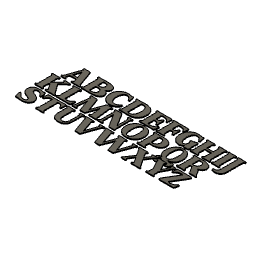
alphabet v02 (Autodesk Fusion 360 design; units mm, degrees)
Autodesk Fusion 360 part; units mm, degrees
(part 1 of 8)
sketch "Sketch1" plane through (0, 0, 0) normal (0, 0, 1) x (1, 0, 0)
  line L0 (-281.2306, -198.9387) -> (-284.5117, -189.696)
  line L1 (-284.5117, -189.696) -> (-287.7576, -198.9035)
  line L2 (-287.7576, -198.9035) -> (-281.2306, -198.9387)
  spline S0 degree 3 poles (-289.8743, -204.8301) (-290.4035, -206.2765) (-288.1104, -206.2412) (-288.1104, -206.7704) knots 0 0 0 0 1 1 1 1
  spline S1 degree 3 poles (-288.1104, -206.7704) (-288.1104, -207.1937) (-288.4985, -208.0051) (-288.7807, -207.9699) knots 0 0 0 0 1 1 1 1
  spline S2 degree 3 poles (-288.7807, -207.9699) (-289.3099, -207.8993) (-290.3686, -207.864) (-291.4269, -207.864) knots 0 0 0 0 1 1 1 1
  spline S3 degree 3 poles (-291.4269, -207.864) (-292.4852, -207.864) (-293.5436, -207.8993) (-294.0727, -207.9699) knots 0 0 0 0 1 1 1 1
  spline S4 degree 3 poles (-294.0727, -207.9699) (-294.3902, -208.0051) (-294.743, -207.1937) (-294.743, -206.7704) knots 0 0 0 0 1 1 1 1
  spline S5 degree 3 poles (-294.743, -206.7704) (-294.743, -206.2412) (-293.1555, -206.2412) (-292.6616, -204.8301) knots 0 0 0 0 1 1 1 1
  line L3 (-292.6616, -204.8301) -> (-286.0992, -186.4151)
  spline S6 degree 3 poles (-286.0992, -186.4151) (-286.699, -185.9565) (-287.4045, -185.7801) (-287.4045, -185.4274) knots 0 0 0 0 1 1 1 1
  spline S7 degree 3 poles (-287.4045, -185.4274) (-287.4045, -185.004) (-287.0168, -184.2244) (-286.7346, -184.2632) knots 0 0 0 0 1 1 1 1
  spline S8 degree 3 poles (-286.7346, -184.2632) (-284.2295, -184.4749) (-281.5484, -184.2632) (-280.3486, -184.2632) knots 0 0 0 0 1 1 1 1
  spline S9 degree 3 poles (-280.3486, -184.2632) (-279.1492, -184.2632) (-278.7964, -184.4749) (-278.5847, -185.0746) knots 0 0 0 0 1 1 1 1
  line L4 (-278.5847, -185.0746) -> (-271.5641, -204.8301)
  spline S10 degree 3 poles (-271.5641, -204.8301) (-271.0702, -206.2765) (-269.4827, -206.2412) (-269.4827, -206.7704) knots 0 0 0 0 1 1 1 1
  spline S11 degree 3 poles (-269.4827, -206.7704) (-269.4827, -207.1937) (-269.8355, -207.9699) (-270.1174, -207.9699) knots 0 0 0 0 1 1 1 1
  spline S12 degree 3 poles (-270.1174, -207.9699) (-271.5288, -207.8993) (-273.3633, -207.864) (-275.1981, -207.864) knots 0 0 0 0 1 1 1 1
  spline S13 degree 3 poles (-275.1981, -207.864) (-277.0325, -207.864) (-278.8317, -207.8993) (-280.2428, -207.9699) knots 0 0 0 0 1 1 1 1
  spline S14 degree 3 poles (-280.2428, -207.9699) (-280.525, -207.9699) (-280.9134, -207.1937) (-280.9134, -206.7704) knots 0 0 0 0 1 1 1 1
  spline S15 degree 3 poles (-280.9134, -206.7704) (-280.9134, -206.2412) (-278.6553, -206.2765) (-279.1492, -204.8301) knots 0 0 0 0 1 1 1 1
  line L5 (-279.1492, -204.8301) -> (-280.3842, -201.4082)
  line L6 (-280.3842, -201.4082) -> (-288.6749, -201.4787)
  line L7 (-288.6749, -201.4787) -> (-289.8743, -204.8301)
  spline S16 degree 3 poles (-259.2536, -204.7243) (-259.2536, -205.571) (-257.4897, -205.5357) (-256.8194, -205.5357) knots 0 0 0 0 1 1 1 1
  spline S17 degree 3 poles (-256.8194, -205.5357) (-253.2916, -205.5357) (-251.351, -204.0187) (-251.351, -201.1965) knots 0 0 0 0 1 1 1 1
  spline S18 degree 3 poles (-251.351, -201.1965) (-251.351, -198.3743) (-253.256, -196.8221) (-256.6787, -196.8221) knots 0 0 0 0 1 1 1 1
  line L8 (-256.6787, -196.8221) -> (-259.2536, -196.8221)
  line L9 (-259.2536, -196.8221) -> (-259.2536, -204.7243)
  spline S19 degree 3 poles (-256.9605, -194.3526) (-254.103, -194.3526) (-252.4093, -192.9415) (-252.4093, -190.5426) knots 0 0 0 0 1 1 1 1
  spline S20 degree 3 poles (-252.4093, -190.5426) (-252.4093, -188.179) (-254.103, -186.7326) (-256.9605, -186.7326) knots 0 0 0 0 1 1 1 1
  spline S21 degree 3 poles (-256.9605, -186.7326) (-258.76, -186.7326) (-259.2536, -186.6974) (-259.2536, -187.544) knots 0 0 0 0 1 1 1 1
  line L10 (-259.2536, -187.544) -> (-259.2536, -194.3526)
  line L11 (-259.2536, -194.3526) -> (-256.9605, -194.3526)
  spline S22 degree 3 poles (-243.6248, -201.3729) (-243.6248, -205.7121) (-247.5763, -208.0051) (-255.1614, -208.0051) knots 0 0 0 0 1 1 1 1
  spline S23 degree 3 poles (-255.1614, -208.0051) (-258.8659, -208.0051) (-260.4883, -207.8993) (-262.9934, -207.8993) knots 0 0 0 0 1 1 1 1
  spline S24 degree 3 poles (-262.9934, -207.8993) (-264.5456, -207.8993) (-266.2393, -207.9346) (-267.6504, -208.0051) knots 0 0 0 0 1 1 1 1
  spline S25 degree 3 poles (-267.6504, -208.0051) (-267.9326, -208.0404) (-268.321, -207.2643) (-268.321, -206.841) knots 0 0 0 0 1 1 1 1
  spline S26 degree 3 poles (-268.321, -206.841) (-268.321, -206.2765) (-266.3804, -206.3824) (-266.3804, -204.9007) knots 0 0 0 0 1 1 1 1
  line L12 (-266.3804, -204.9007) -> (-266.3804, -187.3676)
  spline S27 degree 3 poles (-266.3804, -187.3676) (-266.3804, -185.886) (-268.321, -185.9918) (-268.321, -185.4274) knots 0 0 0 0 1 1 1 1
  spline S28 degree 3 poles (-268.321, -185.4274) (-268.321, -185.004) (-267.9326, -184.2244) (-267.6504, -184.2632) knots 0 0 0 0 1 1 1 1
  spline S29 degree 3 poles (-267.6504, -184.2632) (-266.2393, -184.3337) (-264.5456, -184.369) (-262.9934, -184.369) knots 0 0 0 0 1 1 1 1
  spline S30 degree 3 poles (-262.9934, -184.369) (-260.4883, -184.369) (-258.8659, -184.2632) (-255.1614, -184.2632) knots 0 0 0 0 1 1 1 1
  spline S31 degree 3 poles (-255.1614, -184.2632) (-248.2462, -184.2632) (-244.6832, -186.4857) (-244.6832, -190.2957) knots 0 0 0 0 1 1 1 1
  spline S32 degree 3 poles (-244.6832, -190.2957) (-244.6832, -192.5182) (-245.8826, -194.2115) (-248.2818, -195.3404) knots 0 0 0 0 1 1 1 1
  spline S33 degree 3 poles (-248.2818, -195.3404) (-245.2476, -196.5046) (-243.6248, -198.586) (-243.6248, -201.3729) knots 0 0 0 0 1 1 1 1
  spline S34 degree 3 poles (-220.7302, -201.0201) (-220.5189, -200.7732) (-219.4606, -201.0907) (-219.4606, -201.3729) knots 0 0 0 0 1 1 1 1
  spline S35 degree 3 poles (-219.4606, -201.3729) (-219.4606, -202.5371) (-222.4945, -208.3579) (-229.762, -208.3579) knots 0 0 0 0 1 1 1 1
  spline S36 degree 3 poles (-229.762, -208.3579) (-236.5713, -208.3579) (-241.475, -203.2426) (-241.475, -196.1518) knots 0 0 0 0 1 1 1 1
  spline S37 degree 3 poles (-241.475, -196.1518) (-241.475, -188.9904) (-236.4655, -183.9104) (-229.4445, -183.9104) knots 0 0 0 0 1 1 1 1
  spline S38 degree 3 poles (-229.4445, -183.9104) (-226.622, -183.9104) (-225.3167, -184.616) (-224.1173, -184.616) knots 0 0 0 0 1 1 1 1
  spline S39 degree 3 poles (-224.1173, -184.616) (-223.2353, -184.616) (-222.9531, -184.2632) (-222.3883, -184.2632) knots 0 0 0 0 1 1 1 1
  spline S40 degree 3 poles (-222.3883, -184.2632) (-221.93, -184.2632) (-221.6478, -184.6865) (-221.4714, -185.3568) knots 0 0 0 0 1 1 1 1
  spline S41 degree 3 poles (-221.4714, -185.3568) (-221.33, -185.886) (-220.5539, -190.3662) (-220.5539, -190.6485) knots 0 0 0 0 1 1 1 1
  spline S42 degree 3 poles (-220.5539, -190.6485) (-220.5539, -190.9307) (-221.33, -191.6715) (-221.7536, -191.6715) knots 0 0 0 0 1 1 1 1
  spline S43 degree 3 poles (-221.7536, -191.6715) (-222.3883, -191.6715) (-224.1525, -186.4504) (-228.4215, -186.4504) knots 0 0 0 0 1 1 1 1
  spline S44 degree 3 poles (-228.4215, -186.4504) (-231.7376, -186.4504) (-233.7135, -189.6254) (-233.7135, -194.9171) knots 0 0 0 0 1 1 1 1
  spline S45 degree 3 poles (-233.7135, -194.9171) (-233.7135, -200.9143) (-231.1735, -204.3715) (-226.9398, -204.3715) knots 0 0 0 0 1 1 1 1
  spline S46 degree 3 poles (-226.9398, -204.3715) (-224.6464, -204.3715) (-222.812, -203.3485) (-220.7302, -201.0201) knots 0 0 0 0 1 1 1 1
  spline S47 degree 3 poles (-206.8319, -186.7326) (-208.5958, -186.7326) (-209.1249, -186.6621) (-209.1249, -187.544) knots 0 0 0 0 1 1 1 1
  line L13 (-209.1249, -187.544) -> (-209.1249, -204.689)
  spline S48 degree 3 poles (-209.1249, -204.689) (-209.1249, -205.571) (-207.3258, -205.5004) (-206.7962, -205.5004) knots 0 0 0 0 1 1 1 1
  spline S49 degree 3 poles (-206.7962, -205.5004) (-202.7746, -205.5004) (-200.5874, -202.3607) (-200.5874, -196.1165) knots 0 0 0 0 1 1 1 1
  spline S50 degree 3 poles (-200.5874, -196.1165) (-200.5874, -189.8724) (-202.7746, -186.7326) (-206.8319, -186.7326) knots 0 0 0 0 1 1 1 1
  spline S51 degree 3 poles (-212.8294, -207.8993) (-214.3817, -207.8993) (-216.1103, -207.9346) (-217.5214, -208.0051) knots 0 0 0 0 1 1 1 1
  spline S52 degree 3 poles (-217.5214, -208.0051) (-217.8036, -208.0051) (-218.1564, -207.2643) (-218.1564, -206.841) knots 0 0 0 0 1 1 1 1
  spline S53 degree 3 poles (-218.1564, -206.841) (-218.1564, -206.2765) (-216.2514, -206.3824) (-216.2514, -204.8654) knots 0 0 0 0 1 1 1 1
  line L14 (-216.2514, -204.8654) -> (-216.2514, -187.3676)
  spline S54 degree 3 poles (-216.2514, -187.3676) (-216.2514, -185.886) (-218.192, -185.9918) (-218.192, -185.4274) knots 0 0 0 0 1 1 1 1
  spline S55 degree 3 poles (-218.192, -185.4274) (-218.192, -185.004) (-217.8036, -184.2244) (-217.5214, -184.2632) knots 0 0 0 0 1 1 1 1
  spline S56 degree 3 poles (-217.5214, -184.2632) (-216.1103, -184.3337) (-214.4169, -184.369) (-212.8294, -184.369) knots 0 0 0 0 1 1 1 1
  spline S57 degree 3 poles (-212.8294, -184.369) (-210.3596, -184.369) (-208.9133, -184.2632) (-205.2087, -184.2632) knots 0 0 0 0 1 1 1 1
  spline S58 degree 3 poles (-205.2087, -184.2632) (-197.8001, -184.2632) (-192.8259, -189.0257) (-192.8259, -196.1518) knots 0 0 0 0 1 1 1 1
  spline S59 degree 3 poles (-192.8259, -196.1518) (-192.8259, -203.2779) (-197.7648, -208.0051) (-205.2087, -208.0051) knots 0 0 0 0 1 1 1 1
  spline S60 degree 3 poles (-205.2087, -208.0051) (-208.9133, -207.9699) (-210.3596, -207.8993) (-212.8294, -207.8993) knots 0 0 0 0 1 1 1 1
  line L15 (-182.4916, -194.4232) -> (-180.0222, -194.3526)
  spline S61 degree 3 poles (-180.0222, -194.3526) (-177.1294, -194.2821) (-177.3411, -190.6485) (-176.2827, -190.6485) knots 0 0 0 0 1 1 1 1
  spline S62 degree 3 poles (-176.2827, -190.6485) (-175.8594, -190.6485) (-175.0833, -191.0365) (-175.0833, -191.3187) knots 0 0 0 0 1 1 1 1
  spline S63 degree 3 poles (-175.0833, -191.3187) (-175.2597, -194.2115) (-175.2597, -197.1043) (-175.0833, -199.9971) knots 0 0 0 0 1 1 1 1
  spline S64 degree 3 poles (-175.0833, -199.9971) (-175.0833, -200.2793) (-175.8594, -200.6674) (-176.2827, -200.6674) knots 0 0 0 0 1 1 1 1
  spline S65 degree 3 poles (-176.2827, -200.6674) (-177.3411, -200.6674) (-177.1294, -197.0337) (-180.0222, -196.9632) knots 0 0 0 0 1 1 1 1
  line L16 (-180.0222, -196.9632) -> (-182.4916, -196.8926)
  line L17 (-182.4916, -196.8926) -> (-182.4916, -204.2657)
  spline S66 degree 3 poles (-182.4916, -204.2657) (-182.4916, -205.1829) (-182.1036, -205.4299) (-179.9163, -205.4299) knots 0 0 0 0 1 1 1 1
  spline S67 degree 3 poles (-179.9163, -205.4299) (-173.5311, -205.4299) (-172.508, -201.3024) (-171.8377, -201.3024) knots 0 0 0 0 1 1 1 1
  spline S68 degree 3 poles (-171.8377, -201.3024) (-171.4144, -201.3024) (-170.6383, -201.6551) (-170.6383, -201.9374) knots 0 0 0 0 1 1 1 1
  spline S69 degree 3 poles (-170.6383, -201.9374) (-170.6383, -202.2196) (-171.5908, -206.4529) (-171.7319, -206.9821) knots 0 0 0 0 1 1 1 1
  spline S70 degree 3 poles (-171.7319, -206.9821) (-171.9788, -207.7935) (-172.2611, -208.0404) (-173.0019, -208.0051) knots 0 0 0 0 1 1 1 1
  spline S71 degree 3 poles (-173.0019, -208.0051) (-175.4713, -207.9346) (-178.6816, -207.8993) (-181.9272, -207.8993) knots 0 0 0 0 1 1 1 1
  spline S72 degree 3 poles (-181.9272, -207.8993) (-185.1371, -207.8993) (-188.3827, -207.9346) (-190.8524, -208.0051) knots 0 0 0 0 1 1 1 1
  spline S73 degree 3 poles (-190.8524, -208.0051) (-191.1696, -208.0051) (-191.5224, -207.2643) (-191.5224, -206.841) knots 0 0 0 0 1 1 1 1
  spline S74 degree 3 poles (-191.5224, -206.841) (-191.5224, -206.2765) (-189.6174, -206.3824) (-189.6174, -204.9007) knots 0 0 0 0 1 1 1 1
  line L18 (-189.6174, -204.9007) -> (-189.6174, -187.4029)
  spline S75 degree 3 poles (-189.6174, -187.4029) (-189.6174, -185.886) (-191.5224, -185.9918) (-191.5224, -185.4626) knots 0 0 0 0 1 1 1 1
  spline S76 degree 3 poles (-191.5224, -185.4626) (-191.5224, -185.0393) (-191.1696, -184.2632) (-190.8524, -184.2632) knots 0 0 0 0 1 1 1 1
  spline S77 degree 3 poles (-190.8524, -184.2632) (-188.5238, -184.3337) (-185.3135, -184.369) (-182.0683, -184.369) knots 0 0 0 0 1 1 1 1
  spline S78 degree 3 poles (-182.0683, -184.369) (-178.4347, -184.369) (-174.7658, -184.3337) (-172.1552, -184.2632) knots 0 0 0 0 1 1 1 1
  spline S79 degree 3 poles (-172.1552, -184.2632) (-171.4497, -184.2244) (-171.0616, -184.4396) (-171.0616, -185.0746) knots 0 0 0 0 1 1 1 1
  spline S80 degree 3 poles (-171.0616, -185.0746) (-171.0616, -185.8507) (-171.5908, -190.0135) (-171.5908, -190.2957) knots 0 0 0 0 1 1 1 1
  spline S81 degree 3 poles (-171.5908, -190.2957) (-171.5908, -190.5779) (-172.3316, -190.966) (-172.7549, -190.966) knots 0 0 0 0 1 1 1 1
  spline S82 degree 3 poles (-172.7549, -190.966) (-173.4252, -190.966) (-173.5311, -186.8385) (-179.9163, -186.8385) knots 0 0 0 0 1 1 1 1
  spline S83 degree 3 poles (-179.9163, -186.8385) (-182.033, -186.8385) (-182.4916, -186.7679) (-182.4916, -187.6146) knots 0 0 0 0 1 1 1 1
  line L19 (-182.4916, -187.6146) -> (-182.4916, -194.4232)
  line L20 (-160.443, -195.1287) -> (-157.9736, -195.0582)
  spline S84 degree 3 poles (-157.9736, -195.0582) (-155.0808, -194.9876) (-155.2924, -191.354) (-154.2341, -191.354) knots 0 0 0 0 1 1 1 1
  spline S85 degree 3 poles (-154.2341, -191.354) (-153.8108, -191.354) (-153.0347, -191.7421) (-153.0347, -192.0243) knots 0 0 0 0 1 1 1 1
  spline S86 degree 3 poles (-153.0347, -192.0243) (-153.2111, -194.9171) (-153.2111, -197.8099) (-153.0347, -200.7026) knots 0 0 0 0 1 1 1 1
  spline S87 degree 3 poles (-153.0347, -200.7026) (-153.0347, -200.9849) (-153.8108, -201.3729) (-154.2341, -201.3729) knots 0 0 0 0 1 1 1 1
  spline S88 degree 3 poles (-154.2341, -201.3729) (-155.2924, -201.3729) (-155.0808, -197.7393) (-157.9736, -197.6687) knots 0 0 0 0 1 1 1 1
  line L21 (-157.9736, -197.6687) -> (-160.443, -197.5982)
  line L22 (-160.443, -197.5982) -> (-160.443, -204.8654)
  spline S89 degree 3 poles (-160.443, -204.8654) (-160.443, -206.3824) (-158.5027, -206.2765) (-158.5027, -206.8057) knots 0 0 0 0 1 1 1 1
  spline S90 degree 3 poles (-158.5027, -206.8057) (-158.5027, -207.2643) (-158.8908, -208.0051) (-159.173, -208.0051) knots 0 0 0 0 1 1 1 1
  spline S91 degree 3 poles (-159.173, -208.0051) (-160.5488, -207.9346) (-162.2774, -207.8993) (-163.9708, -207.8993) knots 0 0 0 0 1 1 1 1
  spline S92 degree 3 poles (-163.9708, -207.8993) (-165.6994, -207.8993) (-167.3927, -207.9346) (-168.8038, -208.0051) knots 0 0 0 0 1 1 1 1
  spline S93 degree 3 poles (-168.8038, -208.0051) (-169.1213, -208.0051) (-169.4741, -207.2643) (-169.4741, -206.841) knots 0 0 0 0 1 1 1 1
  spline S94 degree 3 poles (-169.4741, -206.841) (-169.4741, -206.2765) (-167.5691, -206.3824) (-167.5691, -204.8654) knots 0 0 0 0 1 1 1 1
  line L23 (-167.5691, -204.8654) -> (-167.5691, -187.4029)
  spline S95 degree 3 poles (-167.5691, -187.4029) (-167.5691, -185.886) (-169.4741, -185.9918) (-169.4741, -185.4626) knots 0 0 0 0 1 1 1 1
  spline S96 degree 3 poles (-169.4741, -185.4626) (-169.4741, -185.0393) (-169.1213, -184.2632) (-168.8038, -184.2632) knots 0 0 0 0 1 1 1 1
  spline S97 degree 3 poles (-168.8038, -184.2632) (-166.4755, -184.3337) (-163.2652, -184.369) (-160.0197, -184.369) knots 0 0 0 0 1 1 1 1
  spline S98 degree 3 poles (-160.0197, -184.369) (-156.3861, -184.369) (-152.7172, -184.3337) (-150.1066, -184.2632) knots 0 0 0 0 1 1 1 1
  spline S99 degree 3 poles (-150.1066, -184.2632) (-149.4011, -184.2244) (-148.9777, -184.4396) (-148.9777, -185.0746) knots 0 0 0 0 1 1 1 1
  spline S100 degree 3 poles (-148.9777, -185.0746) (-148.9777, -185.8507) (-149.5422, -190.0135) (-149.5422, -190.2957) knots 0 0 0 0 1 1 1 1
  spline S101 degree 3 poles (-149.5422, -190.2957) (-149.5422, -190.5779) (-150.283, -190.966) (-150.7063, -190.966) knots 0 0 0 0 1 1 1 1
  spline S102 degree 3 poles (-150.7063, -190.966) (-151.3766, -190.966) (-151.4824, -186.8385) (-157.8677, -186.8385) knots 0 0 0 0 1 1 1 1
  spline S103 degree 3 poles (-157.8677, -186.8385) (-159.9844, -186.8385) (-160.443, -186.7679) (-160.443, -187.6146) knots 0 0 0 0 1 1 1 1
  line L24 (-160.443, -187.6146) -> (-160.443, -195.1287)
  spline S104 degree 3 poles (-149.2599, -196.1518) (-149.2599, -188.9904) (-144.2858, -183.9104) (-137.2302, -183.9104) knots 0 0 0 0 1 1 1 1
  spline S105 degree 3 poles (-137.2302, -183.9104) (-134.408, -183.9104) (-132.7499, -184.616) (-131.5505, -184.616) knots 0 0 0 0 1 1 1 1
  spline S106 degree 3 poles (-131.5505, -184.616) (-130.6686, -184.616) (-130.3863, -184.2632) (-129.8219, -184.2632) knots 0 0 0 0 1 1 1 1
  spline S107 degree 3 poles (-129.8219, -184.2632) (-129.3633, -184.2632) (-129.0811, -184.6865) (-128.9047, -185.3568) knots 0 0 0 0 1 1 1 1
  spline S108 degree 3 poles (-128.9047, -185.3568) (-128.7636, -185.886) (-127.9874, -190.3662) (-127.9874, -190.6485) knots 0 0 0 0 1 1 1 1
  spline S109 degree 3 poles (-127.9874, -190.6485) (-127.9874, -190.9307) (-128.7636, -191.6715) (-129.1869, -191.6715) knots 0 0 0 0 1 1 1 1
  spline S110 degree 3 poles (-129.1869, -191.6715) (-129.8572, -191.6715) (-131.9386, -186.4504) (-136.2072, -186.4504) knots 0 0 0 0 1 1 1 1
  spline S111 degree 3 poles (-136.2072, -186.4504) (-139.5586, -186.4504) (-141.4988, -189.6607) (-141.4988, -195.2346) knots 0 0 0 0 1 1 1 1
  spline S112 degree 3 poles (-141.4988, -195.2346) (-141.4988, -200.8085) (-139.5586, -204.3715) (-136.7011, -204.3715) knots 0 0 0 0 1 1 1 1
  spline S113 degree 3 poles (-136.7011, -204.3715) (-134.7961, -204.3715) (-133.5261, -202.8546) (-133.5261, -200.5615) knots 0 0 0 0 1 1 1 1
  line L25 (-133.5261, -200.5615) -> (-133.5261, -199.1857)
  spline S114 degree 3 poles (-133.5261, -199.1857) (-133.5261, -197.6687) (-135.1136, -197.7746) (-135.1136, -197.2454) knots 0 0 0 0 1 1 1 1
  spline S115 degree 3 poles (-135.1136, -197.2454) (-135.1136, -196.8221) (-134.7255, -196.0812) (-134.4433, -196.046) knots 0 0 0 0 1 1 1 1
  spline S116 degree 3 poles (-134.4433, -196.046) (-130.4922, -195.6932) (-128.3049, -194.3879) (-127.7405, -194.3879) knots 0 0 0 0 1 1 1 1
  spline S117 degree 3 poles (-127.7405, -194.3879) (-127.3172, -194.3879) (-126.5411, -194.776) (-126.5763, -195.0582) knots 0 0 0 0 1 1 1 1
  spline S118 degree 3 poles (-126.5763, -195.0582) (-127.2819, -201.761) (-127.1055, -204.9712) (-126.4352, -206.841) knots 0 0 0 0 1 1 1 1
  spline S119 degree 3 poles (-126.4352, -206.841) (-126.2588, -207.229) (-126.788, -208.0404) (-127.0702, -208.0051) knots 0 0 0 0 1 1 1 1
  spline S120 degree 3 poles (-127.0702, -208.0051) (-128.1286, -207.9346) (-128.9047, -207.8993) (-129.7161, -207.8993) knots 0 0 0 0 1 1 1 1
  spline S121 degree 3 poles (-129.7161, -207.8993) (-130.4922, -207.8993) (-131.3036, -207.9346) (-132.3619, -208.0051) knots 0 0 0 0 1 1 1 1
  spline S122 degree 3 poles (-132.3619, -208.0051) (-132.7852, -208.0404) (-133.5261, -207.6171) (-133.5261, -207.3349) knots 0 0 0 0 1 1 1 1
  line L26 (-133.5261, -207.3349) -> (-133.5261, -205.959)
  spline S123 degree 3 poles (-133.5261, -205.959) (-134.9372, -207.3349) (-136.7363, -208.3579) (-138.3238, -208.3579) knots 0 0 0 0 1 1 1 1
  spline S124 degree 3 poles (-138.3238, -208.3579) (-144.6738, -208.3579) (-149.2599, -203.2426) (-149.2599, -196.1518) knots 0 0 0 0 1 1 1 1
  line L27 (-115.8872, -194.141) -> (-107.4205, -194.141)
  line L28 (-107.4205, -194.141) -> (-107.4205, -187.3676)
  spline S125 degree 3 poles (-107.4205, -187.3676) (-107.4205, -185.886) (-109.3255, -185.9918) (-109.3255, -185.4274) knots 0 0 0 0 1 1 1 1
  spline S126 degree 3 poles (-109.3255, -185.4274) (-109.3255, -185.004) (-108.9727, -184.2244) (-108.6905, -184.2632) knots 0 0 0 0 1 1 1 1
  spline S127 degree 3 poles (-108.6905, -184.2632) (-107.2794, -184.3337) (-105.5508, -184.369) (-103.8574, -184.369) knots 0 0 0 0 1 1 1 1
  spline S128 degree 3 poles (-103.8574, -184.369) (-102.1288, -184.369) (-100.4002, -184.3337) (-99.0244, -184.2632) knots 0 0 0 0 1 1 1 1
  spline S129 degree 3 poles (-99.0244, -184.2632) (-98.7422, -184.2244) (-98.3541, -185.004) (-98.3541, -185.4274) knots 0 0 0 0 1 1 1 1
  spline S130 degree 3 poles (-98.3541, -185.4274) (-98.3541, -185.9918) (-100.2944, -185.886) (-100.2944, -187.3676) knots 0 0 0 0 1 1 1 1
  line L29 (-100.2944, -187.3676) -> (-100.2944, -204.8654)
  spline S131 degree 3 poles (-100.2944, -204.8654) (-100.2944, -206.3824) (-98.3541, -206.2765) (-98.3541, -206.841) knots 0 0 0 0 1 1 1 1
  spline S132 degree 3 poles (-98.3541, -206.841) (-98.3541, -207.2643) (-98.7422, -208.0051) (-99.0244, -208.0051) knots 0 0 0 0 1 1 1 1
  spline S133 degree 3 poles (-99.0244, -208.0051) (-100.4002, -207.9346) (-102.1288, -207.8993) (-103.8574, -207.8993) knots 0 0 0 0 1 1 1 1
  spline S134 degree 3 poles (-103.8574, -207.8993) (-105.5508, -207.8993) (-107.2794, -207.9346) (-108.6905, -208.0051) knots 0 0 0 0 1 1 1 1
  spline S135 degree 3 poles (-108.6905, -208.0051) (-108.9727, -208.0051) (-109.3255, -207.2643) (-109.3255, -206.841) knots 0 0 0 0 1 1 1 1
  spline S136 degree 3 poles (-109.3255, -206.841) (-109.3255, -206.2765) (-107.4205, -206.3824) (-107.4205, -204.8654) knots 0 0 0 0 1 1 1 1
  line L30 (-107.4205, -204.8654) -> (-107.4205, -196.7868)
  line L31 (-107.4205, -196.7868) -> (-115.8872, -196.7868)
  line L32 (-115.8872, -196.7868) -> (-115.8872, -204.8654)
  spline S137 degree 3 poles (-115.8872, -204.8654) (-115.8872, -206.3824) (-113.9469, -206.2765) (-113.9469, -206.841) knots 0 0 0 0 1 1 1 1
  spline S138 degree 3 poles (-113.9469, -206.841) (-113.9469, -207.2643) (-114.3349, -208.0051) (-114.6172, -208.0051) knots 0 0 0 0 1 1 1 1
  spline S139 degree 3 poles (-114.6172, -208.0051) (-115.993, -207.9346) (-117.7216, -207.8993) (-119.4149, -207.8993) knots 0 0 0 0 1 1 1 1
  spline S140 degree 3 poles (-119.4149, -207.8993) (-121.1436, -207.8993) (-122.8369, -207.9346) (-124.248, -208.0051) knots 0 0 0 0 1 1 1 1
  spline S141 degree 3 poles (-124.248, -208.0051) (-124.5655, -208.0051) (-124.9183, -207.2643) (-124.9183, -206.841) knots 0 0 0 0 1 1 1 1
  spline S142 degree 3 poles (-124.9183, -206.841) (-124.9183, -206.2765) (-123.0133, -206.3824) (-123.0133, -204.8654) knots 0 0 0 0 1 1 1 1
  line L33 (-123.0133, -204.8654) -> (-123.0133, -187.3676)
  spline S143 degree 3 poles (-123.0133, -187.3676) (-123.0133, -185.886) (-124.9183, -185.9918) (-124.9183, -185.4274) knots 0 0 0 0 1 1 1 1
  spline S144 degree 3 poles (-124.9183, -185.4274) (-124.9183, -185.004) (-124.5655, -184.2244) (-124.248, -184.2632) knots 0 0 0 0 1 1 1 1
  spline S145 degree 3 poles (-124.248, -184.2632) (-122.8369, -184.3337) (-121.1436, -184.369) (-119.4149, -184.369) knots 0 0 0 0 1 1 1 1
  spline S146 degree 3 poles (-119.4149, -184.369) (-117.7216, -184.369) (-115.993, -184.3337) (-114.6172, -184.2632) knots 0 0 0 0 1 1 1 1
  spline S147 degree 3 poles (-114.6172, -184.2632) (-114.3349, -184.2244) (-113.9469, -185.004) (-113.9469, -185.4274) knots 0 0 0 0 1 1 1 1
  spline S148 degree 3 poles (-113.9469, -185.4274) (-113.9469, -185.9565) (-115.8872, -185.8507) (-115.8872, -187.3676) knots 0 0 0 0 1 1 1 1
  line L34 (-115.8872, -187.3676) -> (-115.8872, -194.141)
  spline S149 degree 3 poles (-87.8766, -204.8654) (-87.8766, -206.3824) (-85.9363, -206.2765) (-85.9363, -206.8057) knots 0 0 0 0 1 1 1 1
  spline S150 degree 3 poles (-85.9363, -206.8057) (-85.9363, -207.2643) (-86.3244, -208.0051) (-86.6066, -208.0051) knots 0 0 0 0 1 1 1 1
  spline S151 degree 3 poles (-86.6066, -208.0051) (-87.9824, -207.9346) (-89.7111, -207.8993) (-91.4397, -207.8993) knots 0 0 0 0 1 1 1 1
  spline S152 degree 3 poles (-91.4397, -207.8993) (-93.1683, -207.8993) (-94.8651, -207.9346) (-96.2762, -208.0051) knots 0 0 0 0 1 1 1 1
  spline S153 degree 3 poles (-96.2762, -208.0051) (-96.5549, -208.0051) (-96.9077, -207.2643) (-96.9077, -206.841) knots 0 0 0 0 1 1 1 1
  spline S154 degree 3 poles (-96.9077, -206.841) (-96.9077, -206.2765) (-95.0027, -206.3824) (-95.0027, -204.8654) knots 0 0 0 0 1 1 1 1
  line L35 (-95.0027, -204.8654) -> (-95.0027, -187.3676)
  spline S155 degree 3 poles (-95.0027, -187.3676) (-95.0027, -185.886) (-96.9077, -185.9565) (-96.9077, -185.4274) knots 0 0 0 0 1 1 1 1
  spline S156 degree 3 poles (-96.9077, -185.4274) (-96.9077, -185.004) (-96.5549, -184.2244) (-96.2762, -184.2632) knots 0 0 0 0 1 1 1 1
  spline S157 degree 3 poles (-96.2762, -184.2632) (-94.8651, -184.3337) (-93.1683, -184.369) (-91.4397, -184.369) knots 0 0 0 0 1 1 1 1
  spline S158 degree 3 poles (-91.4397, -184.369) (-89.7111, -184.369) (-87.9824, -184.3337) (-86.6066, -184.2632) knots 0 0 0 0 1 1 1 1
  spline S159 degree 3 poles (-86.6066, -184.2632) (-86.3244, -184.2244) (-85.9363, -185.004) (-85.9363, -185.4274) knots 0 0 0 0 1 1 1 1
  spline S160 degree 3 poles (-85.9363, -185.4274) (-85.9363, -185.9565) (-87.8766, -185.886) (-87.8766, -187.3676) knots 0 0 0 0 1 1 1 1
  line L36 (-87.8766, -187.3676) -> (-87.8766, -204.8654)
  spline S161 degree 3 poles (-83.2587, -216.119) (-85.9046, -216.119) (-87.8449, -215.4487) (-88.3035, -214.9901) knots 0 0 0 0 1 1 1 1
  spline S162 degree 3 poles (-88.3035, -214.9901) (-88.5151, -214.7785) (-87.9507, -213.4732) (-87.6332, -213.4732) knots 0 0 0 0 1 1 1 1
  spline S163 degree 3 poles (-87.6332, -213.4732) (-84.1054, -213.4732) (-82.5885, -212.2385) (-82.5885, -207.9699) knots 0 0 0 0 1 1 1 1
  line L37 (-82.5885, -207.9699) -> (-82.5885, -187.4029)
  spline S164 degree 3 poles (-82.5885, -187.4029) (-82.5885, -185.886) (-84.4935, -185.9918) (-84.4935, -185.4626) knots 0 0 0 0 1 1 1 1
  spline S165 degree 3 poles (-84.4935, -185.4626) (-84.4935, -185.0393) (-84.1407, -184.2632) (-83.8585, -184.2632) knots 0 0 0 0 1 1 1 1
  spline S166 degree 3 poles (-83.8585, -184.2632) (-82.4474, -184.3337) (-80.7187, -184.369) (-79.0254, -184.369) knots 0 0 0 0 1 1 1 1
  spline S167 degree 3 poles (-79.0254, -184.369) (-77.2968, -184.369) (-75.5647, -184.3337) (-74.1924, -184.2632) knots 0 0 0 0 1 1 1 1
  spline S168 degree 3 poles (-74.1924, -184.2632) (-73.9066, -184.2632) (-73.5221, -185.0393) (-73.5221, -185.4626) knots 0 0 0 0 1 1 1 1
  spline S169 degree 3 poles (-73.5221, -185.4626) (-73.5221, -185.9918) (-75.4624, -185.886) (-75.4624, -187.4029) knots 0 0 0 0 1 1 1 1
  line L38 (-75.4624, -187.4029) -> (-75.4624, -207.6524)
  spline S170 degree 3 poles (-75.4624, -207.6524) (-75.4624, -213.4026) (-78.0729, -216.119) (-83.2587, -216.119) knots 0 0 0 0 1 1 1 1
  line L39 (-63.0446, -195.6932) -> (-54.4368, -187.4735)
  spline S171 degree 3 poles (-54.4368, -187.4735) (-53.3785, -186.4151) (-55.7774, -186.0271) (-55.7774, -185.4626) knots 0 0 0 0 1 1 1 1
  spline S172 degree 3 poles (-55.7774, -185.4626) (-55.7774, -185.0393) (-55.2835, -184.2632) (-55.0012, -184.2985) knots 0 0 0 0 1 1 1 1
  spline S173 degree 3 poles (-55.0012, -184.2985) (-54.2957, -184.369) (-52.9199, -184.4008) (-51.544, -184.4008) knots 0 0 0 0 1 1 1 1
  spline S174 degree 3 poles (-51.544, -184.4008) (-50.2, -184.4008) (-48.8276, -184.369) (-48.1186, -184.2985) knots 0 0 0 0 1 1 1 1
  spline S175 degree 3 poles (-48.1186, -184.2985) (-47.8363, -184.2632) (-47.4483, -185.0393) (-47.4483, -185.4626) knots 0 0 0 0 1 1 1 1
  spline S176 degree 3 poles (-47.4483, -185.4626) (-47.4483, -186.0271) (-49.4591, -186.4504) (-50.5915, -187.4382) knots 0 0 0 0 1 1 1 1
  line L40 (-50.5915, -187.4382) -> (-56.4476, -192.8357)
  line L41 (-56.4476, -192.8357) -> (-47.8011, -204.8654)
  spline S177 degree 3 poles (-47.8011, -204.8654) (-46.9191, -206.1001) (-45.1905, -206.2765) (-45.1905, -206.841) knots 0 0 0 0 1 1 1 1
  spline S178 degree 3 poles (-45.1905, -206.841) (-45.1905, -207.2643) (-45.5433, -208.0051) (-45.8255, -208.0051) knots 0 0 0 0 1 1 1 1
  spline S179 degree 3 poles (-45.8255, -208.0051) (-47.2366, -207.9346) (-49.4591, -207.8993) (-51.7204, -207.8993) knots 0 0 0 0 1 1 1 1
  spline S180 degree 3 poles (-51.7204, -207.8993) (-53.9429, -207.8993) (-56.1654, -207.9346) (-57.5765, -208.0051) knots 0 0 0 0 1 1 1 1
  spline S181 degree 3 poles (-57.5765, -208.0051) (-57.8587, -208.0051) (-58.2468, -207.2643) (-58.2468, -206.841) knots 0 0 0 0 1 1 1 1
  spline S182 degree 3 poles (-58.2468, -206.841) (-58.2468, -206.2765) (-55.7774, -206.1001) (-56.6593, -204.8654) knots 0 0 0 0 1 1 1 1
  line L42 (-56.6593, -204.8654) -> (-61.7746, -197.7393)
  line L43 (-61.7746, -197.7393) -> (-63.0446, -198.9035)
  line L44 (-63.0446, -198.9035) -> (-63.0446, -204.8654)
  spline S183 degree 3 poles (-63.0446, -204.8654) (-63.0446, -206.3824) (-61.1043, -206.2765) (-61.1043, -206.841) knots 0 0 0 0 1 1 1 1
  spline S184 degree 3 poles (-61.1043, -206.841) (-61.1043, -207.2643) (-61.4924, -208.0051) (-61.7746, -208.0051) knots 0 0 0 0 1 1 1 1
  spline S185 degree 3 poles (-61.7746, -208.0051) (-63.1504, -207.9346) (-64.879, -207.8993) (-66.6076, -207.8993) knots 0 0 0 0 1 1 1 1
  spline S186 degree 3 poles (-66.6076, -207.8993) (-68.3362, -207.8993) (-70.0296, -207.9346) (-71.4407, -208.0051) knots 0 0 0 0 1 1 1 1
  spline S187 degree 3 poles (-71.4407, -208.0051) (-71.7229, -208.0051) (-72.0757, -207.2643) (-72.0757, -206.841) knots 0 0 0 0 1 1 1 1
  spline S188 degree 3 poles (-72.0757, -206.841) (-72.0757, -206.2765) (-70.1707, -206.3824) (-70.1707, -204.8654) knots 0 0 0 0 1 1 1 1
  line L45 (-70.1707, -204.8654) -> (-70.1707, -187.3676)
  spline S189 degree 3 poles (-70.1707, -187.3676) (-70.1707, -185.886) (-72.0757, -185.9918) (-72.0757, -185.4274) knots 0 0 0 0 1 1 1 1
  spline S190 degree 3 poles (-72.0757, -185.4274) (-72.0757, -185.004) (-71.7229, -184.2244) (-71.4407, -184.2632) knots 0 0 0 0 1 1 1 1
  spline S191 degree 3 poles (-71.4407, -184.2632) (-70.0296, -184.3337) (-68.3362, -184.369) (-66.6076, -184.369) knots 0 0 0 0 1 1 1 1
  spline S192 degree 3 poles (-66.6076, -184.369) (-64.879, -184.369) (-63.1504, -184.3337) (-61.7746, -184.2632) knots 0 0 0 0 1 1 1 1
  spline S193 degree 3 poles (-61.7746, -184.2632) (-61.4924, -184.2244) (-61.1043, -185.004) (-61.1043, -185.4274) knots 0 0 0 0 1 1 1 1
  spline S194 degree 3 poles (-61.1043, -185.4274) (-61.1043, -185.9565) (-63.0446, -185.8507) (-63.0446, -187.3676) knots 0 0 0 0 1 1 1 1
  line L46 (-63.0446, -187.3676) -> (-63.0446, -195.6932)
  spline S195 degree 3 poles (-34.9635, -204.2657) (-34.9635, -205.1829) (-34.5754, -205.3946) (-32.3882, -205.3946) knots 0 0 0 0 1 1 1 1
  spline S196 degree 3 poles (-32.3882, -205.3946) (-27.2376, -205.3946) (-25.8618, -201.3024) (-25.1915, -201.3024) knots 0 0 0 0 1 1 1 1
  spline S197 degree 3 poles (-25.1915, -201.3024) (-24.7682, -201.3024) (-23.9921, -201.6551) (-23.9921, -201.9374) knots 0 0 0 0 1 1 1 1
  spline S198 degree 3 poles (-23.9921, -201.9374) (-23.9921, -202.2196) (-24.9446, -206.4529) (-25.0857, -206.9821) knots 0 0 0 0 1 1 1 1
  spline S199 degree 3 poles (-25.0857, -206.9821) (-25.3326, -207.7935) (-25.6149, -208.0404) (-26.3557, -208.0051) knots 0 0 0 0 1 1 1 1
  spline S200 degree 3 poles (-26.3557, -208.0051) (-28.8251, -207.9346) (-31.8237, -207.8993) (-34.8224, -207.8993) knots 0 0 0 0 1 1 1 1
  spline S201 degree 3 poles (-34.8224, -207.8993) (-37.8562, -207.8993) (-40.8549, -207.9346) (-43.3243, -208.0051) knots 0 0 0 0 1 1 1 1
  spline S202 degree 3 poles (-43.3243, -208.0051) (-43.6418, -208.0051) (-43.9946, -207.2643) (-43.9946, -206.841) knots 0 0 0 0 1 1 1 1
  spline S203 degree 3 poles (-43.9946, -206.841) (-43.9946, -206.2765) (-42.0896, -206.3824) (-42.0896, -204.9007) knots 0 0 0 0 1 1 1 1
  line L47 (-42.0896, -204.9007) -> (-42.0896, -187.3676)
  spline S204 degree 3 poles (-42.0896, -187.3676) (-42.0896, -185.8507) (-43.9946, -185.9918) (-43.9946, -185.4274) knots 0 0 0 0 1 1 1 1
  spline S205 degree 3 poles (-43.9946, -185.4274) (-43.9946, -185.004) (-43.6418, -184.2244) (-43.3243, -184.2632) knots 0 0 0 0 1 1 1 1
  spline S206 degree 3 poles (-43.3243, -184.2632) (-41.9132, -184.3337) (-40.2199, -184.369) (-38.4912, -184.369) knots 0 0 0 0 1 1 1 1
  spline S207 degree 3 poles (-38.4912, -184.369) (-36.7979, -184.369) (-35.0693, -184.3337) (-33.6935, -184.2632) knots 0 0 0 0 1 1 1 1
  spline S208 degree 3 poles (-33.6935, -184.2632) (-33.4112, -184.2244) (-33.0232, -185.004) (-33.0232, -185.4274) knots 0 0 0 0 1 1 1 1
  spline S209 degree 3 poles (-33.0232, -185.4274) (-33.0232, -185.9565) (-34.9635, -185.8507) (-34.9635, -187.3676) knots 0 0 0 0 1 1 1 1
  line L48 (-34.9635, -187.3676) -> (-34.9635, -204.2657)
  spline S210 degree 3 poles (-21.2757, -185.4274) (-21.2757, -185.004) (-20.8876, -184.2244) (-20.6054, -184.2632) knots 0 0 0 0 1 1 1 1
  spline S211 degree 3 poles (-20.6054, -184.2632) (-18.1007, -184.4749) (-15.4196, -184.2632) (-14.2201, -184.2632) knots 0 0 0 0 1 1 1 1
  spline S212 degree 3 poles (-14.2201, -184.2632) (-13.0207, -184.2632) (-12.6679, -184.4749) (-12.421, -185.1099) knots 0 0 0 0 1 1 1 1
  line L49 (-12.421, -185.1099) -> (-6.4237, -201.5846)
  line L50 (-6.4237, -201.5846) -> (-0.4265, -185.1099)
  spline S213 degree 3 poles (-0.4265, -185.1099) (-0.1796, -184.4749) (0.1379, -184.2632) (1.3726, -184.2632) knots 0 0 0 0 1 1 1 1
  spline S214 degree 3 poles (1.3726, -184.2632) (2.5721, -184.2632) (4.9357, -184.4749) (7.4757, -184.2632) knots 0 0 0 0 1 1 1 1
  spline S215 degree 3 poles (7.4757, -184.2632) (7.7579, -184.2244) (8.1107, -185.004) (8.1107, -185.4274) knots 0 0 0 0 1 1 1 1
  spline S216 degree 3 poles (8.1107, -185.4274) (8.1107, -185.9918) (5.8882, -185.9565) (6.0293, -187.4382) knots 0 0 0 0 1 1 1 1
  line L51 (6.0293, -187.4382) -> (7.9343, -204.8654)
  spline S217 degree 3 poles (7.9343, -204.8654) (8.0754, -206.3824) (9.6629, -206.2765) (9.6629, -206.8057) knots 0 0 0 0 1 1 1 1
  spline S218 degree 3 poles (9.6629, -206.8057) (9.6629, -207.229) (9.3101, -208.0404) (9.0279, -208.0051) knots 0 0 0 0 1 1 1 1
  spline S219 degree 3 poles (9.0279, -208.0051) (8.4988, -207.9346) (6.3821, -207.8993) (4.2654, -207.8993) knots 0 0 0 0 1 1 1 1
  spline S220 degree 3 poles (4.2654, -207.8993) (2.184, -207.8993) (0.0674, -207.9346) (-0.4618, -208.0051) knots 0 0 0 0 1 1 1 1
  spline S221 degree 3 poles (-0.4618, -208.0051) (-0.744, -208.0404) (-1.1321, -207.229) (-1.1321, -206.8057) knots 0 0 0 0 1 1 1 1
  spline S222 degree 3 poles (-1.1321, -206.8057) (-1.1321, -206.2765) (0.9493, -206.3824) (0.8082, -204.8654) knots 0 0 0 0 1 1 1 1
  line L52 (0.8082, -204.8654) -> (-0.4971, -193.0474)
  line L53 (-0.4971, -193.0474) -> (-5.9299, -208.0051)
  spline S223 degree 3 poles (-5.9299, -208.0051) (-7.1293, -207.9346) (-8.0112, -207.8993) (-8.8932, -207.8993) knots 0 0 0 0 1 1 1 1
  spline S224 degree 3 poles (-8.8932, -207.8993) (-9.7751, -207.8993) (-10.6571, -207.9346) (-11.8918, -208.0051) knots 0 0 0 0 1 1 1 1
  line L54 (-11.8918, -208.0051) -> (-17.1835, -193.0121)
  line L55 (-17.1835, -193.0121) -> (-18.7357, -204.8654)
  spline S225 degree 3 poles (-18.7357, -204.8654) (-18.9474, -206.3824) (-16.8307, -206.2765) (-16.8307, -206.8057) knots 0 0 0 0 1 1 1 1
  spline S226 degree 3 poles (-16.8307, -206.8057) (-16.8307, -207.229) (-17.1835, -208.0404) (-17.4657, -208.0051) knots 0 0 0 0 1 1 1 1
  spline S227 degree 3 poles (-17.4657, -208.0051) (-17.9949, -207.9346) (-18.9826, -207.8993) (-19.9704, -207.8993) knots 0 0 0 0 1 1 1 1
  spline S228 degree 3 poles (-19.9704, -207.8993) (-20.9582, -207.8993) (-21.946, -207.9346) (-22.4751, -208.0051) knots 0 0 0 0 1 1 1 1
  spline S229 degree 3 poles (-22.4751, -208.0051) (-22.7574, -208.0404) (-23.1454, -207.229) (-23.1454, -206.8057) knots 0 0 0 0 1 1 1 1
  spline S230 degree 3 poles (-23.1454, -206.8057) (-23.1454, -206.2765) (-21.5932, -206.3824) (-21.3815, -204.8654) knots 0 0 0 0 1 1 1 1
  line L56 (-21.3815, -204.8654) -> (-19.159, -187.4029)
  spline S231 degree 3 poles (-19.159, -187.4029) (-18.9826, -185.9212) (-21.2757, -185.9918) (-21.2757, -185.4274) knots 0 0 0 0 1 1 1 1
  spline S232 degree 3 poles (33.4401, -206.841) (33.5813, -207.229) (33.0521, -208.0404) (32.7699, -208.0051) knots 0 0 0 0 1 1 1 1
  spline S233 degree 3 poles (32.7699, -208.0051) (30.2651, -207.7935) (28.3954, -208.0051) (27.2313, -208.0051) knots 0 0 0 0 1 1 1 1
  spline S234 degree 3 poles (27.2313, -208.0051) (25.9613, -208.0051) (25.7496, -207.7229) (25.3968, -207.1937) knots 0 0 0 0 1 1 1 1
  line L57 (25.3968, -207.1937) -> (15.2015, -190.9307)
  line L58 (15.2015, -190.9307) -> (15.2015, -204.8654)
  spline S235 degree 3 poles (15.2015, -204.8654) (15.2015, -206.3824) (17.3182, -206.2765) (17.3182, -206.8057) knots 0 0 0 0 1 1 1 1
  spline S236 degree 3 poles (17.3182, -206.8057) (17.3182, -207.229) (16.9301, -208.0404) (16.6479, -208.0051) knots 0 0 0 0 1 1 1 1
  spline S237 degree 3 poles (16.6479, -208.0051) (16.1188, -207.9346) (15.0957, -207.8993) (14.0726, -207.8993) knots 0 0 0 0 1 1 1 1
  spline S238 degree 3 poles (14.0726, -207.8993) (13.0496, -207.8993) (12.0265, -207.9346) (11.4621, -208.0051) knots 0 0 0 0 1 1 1 1
  spline S239 degree 3 poles (11.4621, -208.0051) (11.1799, -208.0404) (10.8271, -207.2643) (10.8271, -206.841) knots 0 0 0 0 1 1 1 1
  spline S240 degree 3 poles (10.8271, -206.841) (10.8271, -206.2765) (12.5557, -206.3824) (12.5557, -204.8654) knots 0 0 0 0 1 1 1 1
  line L59 (12.5557, -204.8654) -> (12.5557, -187.4382)
  spline S241 degree 3 poles (12.5557, -187.4382) (12.5557, -185.9212) (10.8271, -186.0271) (10.8271, -185.4979) knots 0 0 0 0 1 1 1 1
  spline S242 degree 3 poles (10.8271, -185.4979) (10.8271, -185.0746) (11.1799, -184.2244) (11.4621, -184.2632) knots 0 0 0 0 1 1 1 1
  spline S243 degree 3 poles (11.4621, -184.2632) (14.0021, -184.4749) (17.036, -184.2632) (18.2001, -184.2632) knots 0 0 0 0 1 1 1 1
  spline S244 degree 3 poles (18.2001, -184.2632) (19.4701, -184.2632) (19.6818, -184.5454) (20.0346, -185.1099) knots 0 0 0 0 1 1 1 1
  line L60 (20.0346, -185.1099) -> (30.1946, -201.3024)
  line L61 (30.1946, -201.3024) -> (30.1946, -187.4382)
  spline S245 degree 3 poles (30.1946, -187.4382) (30.1946, -185.9212) (28.0779, -186.0271) (28.0779, -185.4626) knots 0 0 0 0 1 1 1 1
  spline S246 degree 3 poles (28.0779, -185.4626) (28.0779, -185.0393) (28.466, -184.2632) (28.7482, -184.2985) knots 0 0 0 0 1 1 1 1
  spline S247 degree 3 poles (28.7482, -184.2985) (29.2774, -184.369) (30.3004, -184.4008) (31.3235, -184.4008) knots 0 0 0 0 1 1 1 1
  spline S248 degree 3 poles (31.3235, -184.4008) (32.3465, -184.4008) (33.4049, -184.369) (33.934, -184.2985) knots 0 0 0 0 1 1 1 1
  spline S249 degree 3 poles (33.934, -184.2985) (34.2163, -184.2632) (34.569, -185.0393) (34.569, -185.4626) knots 0 0 0 0 1 1 1 1
  spline S250 degree 3 poles (34.569, -185.4626) (34.569, -186.0271) (32.8404, -185.9212) (32.8404, -187.4382) knots 0 0 0 0 1 1 1 1
  line L62 (32.8404, -187.4382) -> (32.8404, -202.0785)
  spline S251 degree 3 poles (32.8404, -202.0785) (32.8404, -204.3362) (33.0521, -205.7826) (33.4401, -206.841) knots 0 0 0 0 1 1 1 1
  spline S252 degree 3 poles (53.1933, -196.152) (53.1933, -189.5199) (51.7141, -186.3799) (48.5727, -186.3799) knots 0 0 0 0 1 1 1 1
  spline S253 degree 3 poles (48.5727, -186.3799) (45.3983, -186.3799) (43.9521, -189.6257) (43.9521, -196.152) knots 0 0 0 0 1 1 1 1
  spline S254 degree 3 poles (43.9521, -196.152) (43.9521, -202.6782) (45.3983, -205.8885) (48.5727, -205.8885) knots 0 0 0 0 1 1 1 1
  spline S255 degree 3 poles (48.5727, -205.8885) (51.747, -205.8885) (53.1933, -202.6782) (53.1933, -196.152) knots 0 0 0 0 1 1 1 1
  spline S256 degree 3 poles (60.9552, -196.152) (60.9552, -203.3838) (55.91, -208.358) (48.5727, -208.358) knots 0 0 0 0 1 1 1 1
  spline S257 degree 3 poles (48.5727, -208.358) (41.2354, -208.358) (36.1901, -203.3838) (36.1901, -196.152) knots 0 0 0 0 1 1 1 1
  spline S258 degree 3 poles (36.1901, -196.152) (36.1901, -188.9201) (41.272, -183.9107) (48.5727, -183.9107) knots 0 0 0 0 1 1 1 1
  spline S259 degree 3 poles (48.5727, -183.9107) (55.877, -183.9107) (60.9552, -188.9201) (60.9552, -196.152) knots 0 0 0 0 1 1 1 1
  line L63 (71.2939, -187.544) -> (71.2939, -197.5275)
  spline S260 degree 3 poles (71.2939, -197.5275) (71.7518, -197.7394) (72.3854, -197.8451) (73.1258, -197.8451) knots 0 0 0 0 1 1 1 1
  spline S261 degree 3 poles (73.1258, -197.8451) (76.3011, -197.8451) (78.4879, -195.8342) (78.4879, -192.2711) knots 0 0 0 0 1 1 1 1
  spline S262 degree 3 poles (78.4879, -192.2711) (78.4879, -188.6378) (76.2667, -186.7326) (73.0914, -186.7326) knots 0 0 0 0 1 1 1 1
  spline S263 degree 3 poles (73.0914, -186.7326) (71.7518, -186.7326) (71.2939, -186.8032) (71.2939, -187.544) knots 0 0 0 0 1 1 1 1
  spline S264 degree 3 poles (71.2939, -204.9006) (71.2939, -206.3822) (73.2326, -206.2765) (73.2326, -206.8409) knots 0 0 0 0 1 1 1 1
  spline S265 degree 3 poles (73.2326, -206.8409) (73.2326, -207.2642) (72.8433, -208.005) (72.5647, -208.005) knots 0 0 0 0 1 1 1 1
  spline S266 degree 3 poles (72.5647, -208.005) (71.187, -207.9347) (69.4581, -207.8992) (67.7292, -207.8992) knots 0 0 0 0 1 1 1 1
  spline S267 degree 3 poles (67.7292, -207.8992) (66.0004, -207.8992) (64.3097, -207.9347) (62.8976, -208.005) knots 0 0 0 0 1 1 1 1
  spline S268 degree 3 poles (62.8976, -208.005) (62.6151, -208.005) (62.2602, -207.2642) (62.2602, -206.8409) knots 0 0 0 0 1 1 1 1
  spline S269 degree 3 poles (62.2602, -206.8409) (62.2602, -206.2765) (64.1685, -206.3822) (64.1685, -204.9006) knots 0 0 0 0 1 1 1 1
  line L64 (64.1685, -204.9006) -> (64.1685, -187.3677)
  spline S270 degree 3 poles (64.1685, -187.3677) (64.1685, -185.8861) (62.222, -185.9918) (62.222, -185.4274) knots 0 0 0 0 1 1 1 1
  spline S271 degree 3 poles (62.222, -185.4274) (62.222, -185.0041) (62.6151, -184.2244) (62.8976, -184.2633) knots 0 0 0 0 1 1 1 1
  spline S272 degree 3 poles (62.8976, -184.2633) (64.3097, -184.3339) (66.0004, -184.369) (67.5537, -184.369) knots 0 0 0 0 1 1 1 1
  spline S273 degree 3 poles (67.5537, -184.369) (70.4466, -184.369) (71.0114, -184.2633) (74.328, -184.2633) knots 0 0 0 0 1 1 1 1
  spline S274 degree 3 poles (74.328, -184.2633) (81.8045, -184.2633) (86.2507, -187.2971) (86.2507, -192.2711) knots 0 0 0 0 1 1 1 1
  spline S275 degree 3 poles (86.2507, -192.2711) (86.2507, -197.2455) (81.7701, -200.385) (74.7134, -200.385) knots 0 0 0 0 1 1 1 1
  spline S276 degree 3 poles (74.7134, -200.385) (73.3395, -200.385) (72.2098, -200.2792) (71.2939, -199.9972) knots 0 0 0 0 1 1 1 1
  line L65 (71.2939, -199.9972) -> (71.2939, -204.9006)
  spline S277 degree 3 poles (105.4075, -196.1516) (105.4075, -189.5194) (103.9264, -186.3799) (100.7849, -186.3799) knots 0 0 0 0 1 1 1 1
  spline S278 degree 3 poles (100.7849, -186.3799) (97.6115, -186.3799) (96.1622, -189.6253) (96.1622, -196.1516) knots 0 0 0 0 1 1 1 1
  spline S279 degree 3 poles (96.1622, -196.1516) (96.1622, -202.6783) (97.6116, -205.8883) (100.7849, -205.8883) knots 0 0 0 0 1 1 1 1
  spline S280 degree 3 poles (100.7849, -205.8883) (103.9622, -205.8883) (105.4075, -202.6783) (105.4075, -196.1516) knots 0 0 0 0 1 1 1 1
  spline S281 degree 3 poles (113.1677, -196.1516) (113.1677, -202.5724) (109.1822, -207.2289) (103.1141, -208.1817) knots 0 0 0 0 1 1 1 1
  spline S282 degree 3 poles (103.1141, -208.1817) (104.7705, -208.64) (106.2517, -209.0282) (107.2391, -209.0282) knots 0 0 0 0 1 1 1 1
  spline S283 degree 3 poles (107.2391, -209.0282) (108.5092, -209.0282) (108.9352, -208.4636) (108.9352, -207.6876) knots 0 0 0 0 1 1 1 1
  spline S284 degree 3 poles (108.9352, -207.6876) (108.9352, -207.6171) (109.1105, -207.5817) (109.3573, -207.5817) knots 0 0 0 0 1 1 1 1
  spline S285 degree 3 poles (109.3573, -207.5817) (110.1695, -207.5817) (111.9692, -208.1463) (111.9692, -210.5802) knots 0 0 0 0 1 1 1 1
  spline S286 degree 3 poles (111.9692, -210.5802) (111.9692, -213.2615) (109.8868, -215.5545) (106.7812, -215.484) knots 0 0 0 0 1 1 1 1
  spline S287 degree 3 poles (106.7812, -215.484) (101.5254, -215.3431) (97.504, -209.0636) (94.9279, -209.0636) knots 0 0 0 0 1 1 1 1
  spline S288 degree 3 poles (94.9279, -209.0636) (93.9404, -209.0636) (93.4109, -209.8042) (93.4109, -210.5452) knots 0 0 0 0 1 1 1 1
  spline S289 degree 3 poles (93.4109, -210.5452) (93.4109, -211.3212) (93.8369, -212.0268) (95.0712, -212.0268) knots 0 0 0 0 1 1 1 1
  spline S290 degree 3 poles (95.0712, -212.0268) (95.987, -212.0268) (96.3772, -211.2858) (96.6559, -211.2858) knots 0 0 0 0 1 1 1 1
  spline S291 degree 3 poles (96.6559, -211.2858) (97.504, -211.2858) (98.6348, -212.5559) (98.6348, -213.6847) knots 0 0 0 0 1 1 1 1
  spline S292 degree 3 poles (98.6348, -213.6847) (98.6348, -215.1667) (96.7993, -216.7541) (94.6452, -216.7541) knots 0 0 0 0 1 1 1 1
  spline S293 degree 3 poles (94.6452, -216.7541) (92.0731, -216.7541) (89.9906, -214.4962) (89.9906, -211.7445) knots 0 0 0 0 1 1 1 1
  spline S294 degree 3 poles (89.9906, -211.7445) (89.9906, -208.9223) (91.6789, -207.3702) (94.6133, -206.9466) knots 0 0 0 0 1 1 1 1
  spline S295 degree 3 poles (94.6133, -206.9466) (90.7671, -204.9713) (88.398, -201.0908) (88.398, -196.1516) knots 0 0 0 0 1 1 1 1
  spline S296 degree 3 poles (88.398, -196.1516) (88.398, -188.9198) (93.4825, -183.9105) (100.7848, -183.9105) knots 0 0 0 0 1 1 1 1
  spline S297 degree 3 poles (100.7848, -183.9105) (108.0871, -183.9105) (113.1677, -188.9198) (113.1677, -196.1516) knots 0 0 0 0 1 1 1 1
  line L66 (123.5029, -186.7678) -> (123.5029, -195.2699)
  spline S298 degree 3 poles (123.5029, -195.2699) (123.5029, -196.1517) (124.669, -196.0812) (125.2334, -196.0812) knots 0 0 0 0 1 1 1 1
  spline S299 degree 3 poles (125.2334, -196.0812) (128.7607, -196.0812) (130.6655, -194.2113) (130.6655, -191.389) knots 0 0 0 0 1 1 1 1
  spline S300 degree 3 poles (130.6655, -191.389) (130.6655, -188.6377) (128.8313, -186.7678) (125.3039, -186.7678) knots 0 0 0 0 1 1 1 1
  line L67 (125.3039, -186.7678) -> (123.5029, -186.7678)
  spline S301 degree 3 poles (116.3736, -187.3675) (116.3736, -185.886) (114.4356, -185.9918) (114.4356, -185.4274) knots 0 0 0 0 1 1 1 1
  spline S302 degree 3 poles (114.4356, -185.4274) (114.4356, -185.0037) (114.8215, -184.2244) (115.1037, -184.263) knots 0 0 0 0 1 1 1 1
  spline S303 degree 3 poles (115.1037, -184.263) (116.5146, -184.3335) (118.2077, -184.3688) (119.7639, -184.3688) knots 0 0 0 0 1 1 1 1
  spline S304 degree 3 poles (119.7639, -184.3688) (122.2704, -184.3688) (122.8348, -184.263) (126.5405, -184.263) knots 0 0 0 0 1 1 1 1
  spline S305 degree 3 poles (126.5405, -184.263) (133.8774, -184.263) (138.4629, -186.9442) (138.4629, -191.4596) knots 0 0 0 0 1 1 1 1
  spline S306 degree 3 poles (138.4629, -191.4596) (138.4629, -194.564) (136.2759, -196.7867) (132.4996, -197.8801) knots 0 0 0 0 1 1 1 1
  spline S307 degree 3 poles (132.4996, -197.8801) (135.2177, -198.8682) (136.3797, -201.9021) (138.1433, -204.8302) knots 0 0 0 0 1 1 1 1
  spline S308 degree 3 poles (138.1433, -204.8302) (138.9194, -206.1353) (140.5793, -206.2764) (140.5793, -206.8055) knots 0 0 0 0 1 1 1 1
  spline S309 degree 3 poles (140.5793, -206.8055) (140.5793, -207.2288) (140.1892, -208.0052) (139.907, -208.0052) knots 0 0 0 0 1 1 1 1
  spline S310 degree 3 poles (139.907, -208.0052) (135.641, -207.7583) (133.6657, -207.9699) (132.4996, -207.9699) knots 0 0 0 0 1 1 1 1
  spline S311 degree 3 poles (132.4996, -207.9699) (130.2421, -207.9699) (131.6199, -207.1582) (130.0305, -204.8302) knots 0 0 0 0 1 1 1 1
  line L68 (130.0305, -204.8302) -> (125.8351, -198.6213)
  line L69 (125.8351, -198.6213) -> (123.5029, -198.6213)
  line L70 (123.5029, -198.6213) -> (123.5029, -204.9008)
  spline S312 degree 3 poles (123.5029, -204.9008) (123.5029, -206.3822) (125.445, -206.2764) (125.445, -206.8408) knots 0 0 0 0 1 1 1 1
  spline S313 degree 3 poles (125.445, -206.8408) (125.445, -207.2641) (125.059, -208.0052) (124.7769, -208.0052) knots 0 0 0 0 1 1 1 1
  spline S314 degree 3 poles (124.7769, -208.0052) (123.3991, -207.9347) (121.6687, -207.8994) (119.9382, -207.8994) knots 0 0 0 0 1 1 1 1
  spline S315 degree 3 poles (119.9382, -207.8994) (118.2077, -207.8994) (116.5146, -207.9347) (115.1037, -208.0052) knots 0 0 0 0 1 1 1 1
  spline S316 degree 3 poles (115.1037, -208.0052) (114.8215, -208.0052) (114.4356, -207.2641) (114.4356, -206.8408) knots 0 0 0 0 1 1 1 1
  spline S317 degree 3 poles (114.4356, -206.8408) (114.4356, -206.2764) (116.3736, -206.3822) (116.3736, -204.9008) knots 0 0 0 0 1 1 1 1
  line L71 (116.3736, -204.9008) -> (116.3736, -187.3675)
  spline S318 degree 3 poles (141.4918, -191.1422) (141.4918, -186.7325) (144.986, -183.9103) (150.4537, -183.9103) knots 0 0 0 0 1 1 1 1
  spline S319 degree 3 poles (150.4537, -183.9103) (153.6275, -183.9103) (154.9347, -184.6159) (156.1691, -184.6159) knots 0 0 0 0 1 1 1 1
  spline S320 degree 3 poles (156.1691, -184.6159) (157.0491, -184.6159) (157.2969, -184.2631) (157.8991, -184.2631) knots 0 0 0 0 1 1 1 1
  spline S321 degree 3 poles (157.8991, -184.2631) (158.3562, -184.2631) (158.6082, -184.6864) (158.7834, -185.3566) knots 0 0 0 0 1 1 1 1
  spline S322 degree 3 poles (158.7834, -185.3566) (158.9585, -185.8859) (159.6975, -190.366) (159.6975, -190.6484) knots 0 0 0 0 1 1 1 1
  spline S323 degree 3 poles (159.6975, -190.6484) (159.6975, -190.9307) (158.9585, -191.6714) (158.5314, -191.6714) knots 0 0 0 0 1 1 1 1
  spline S324 degree 3 poles (158.5314, -191.6714) (157.8607, -191.6714) (155.0756, -186.4502) (150.9108, -186.4502) knots 0 0 0 0 1 1 1 1
  spline S325 degree 3 poles (150.9108, -186.4502) (149.2192, -186.4502) (147.9505, -187.4732) (147.9505, -188.8491) knots 0 0 0 0 1 1 1 1
  spline S326 degree 3 poles (147.9505, -188.8491) (147.9505, -193.2588) (160.4408, -192.518) (160.4408, -201.1258) knots 0 0 0 0 1 1 1 1
  spline S327 degree 3 poles (160.4408, -201.1258) (160.4408, -205.7473) (156.8057, -208.3577) (150.3469, -208.3577) knots 0 0 0 0 1 1 1 1